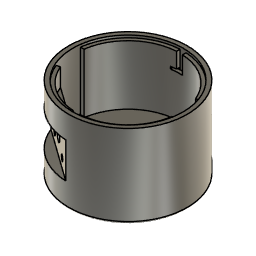
lamp_base v7 (Autodesk Fusion 360 design; units mm, degrees)
Autodesk Fusion 360 part; units mm, degrees
note: some values were not read from the file. Chosen so that the rebuilt part matches the saved one: which face or edge a step refers to. Set by a fixed rule: which sketch regions a step uses.
sketch "Sketch1" plane through (0, 0, 0) normal (0, 0, 1) x (1, 0, 0)
  circle A0 centre (0, 0) radius 50
  constraint coincident A0.centre origin
extrude "Extrude1" add sketch "Sketch1" along normal blind 70
sketch "Sketch2" plane through (0, 0, 0) normal (0, 0, -1) x (1, 0, 0)
  circle A0 centre (0, 0) radius 50
  circle A1 centre (0, 0) radius 40
  dimension "d3" = 80
  constraint coincident A0.centre A1.centre
  measures "d3" diameter of A1
extrude "Extrude2" cut sketch "Sketch2" against normal blind 10 contours A1
sketch "Sketch3" plane through (0, 0, 70) normal (0, 0, 1) x (-1, 0, 0)
  circle A0 centre (0, 0) radius 50
  circle A1 centre (0, 0) radius 46.5
  dimension "d6" = 93
  constraint coincident A0.centre A1.centre
  measures "d6" diameter of A1
extrude "Extrude3" cut sketch "Sketch3" against normal blind 2 contours A1
sketch "Sketch4" plane through (0, 0, 68) normal (0, 0, 1) x (-1, 0, 0)
  circle A0 centre (0, 0) radius 46.5
  circle A1 centre (0, 0) radius 43.5
  dimension "d9" = 87
  constraint coincident A0.centre A1.centre
  measures "d9" diameter of A1
extrude "Extrude4" cut sketch "Sketch4" against normal blind 50 contours A1
sketch "Sketch5" plane through (0, 0, 68) normal (0, 0, 1) x (-1, 0, 0)
  circle A0 centre (0, 0) radius 43.5
  circle A1 centre (0, 0) radius 46.5
  arc A2 (-2.5, -46.4327) -> (2.5, -46.4327) centre (0, 0) ccw
  arc A3 (2.5, 46.4327) -> (-2.5, 46.4327) centre (0, 0) ccw
  line L0 (2.5, 43.4281) -> (-2.5, 43.4281)
  line L1 (2.5, -43.4281) -> (-2.5, -43.4281)
  line L2 (2.5, -46.4327) -> (2.5, -43.4281)
  line L3 (2.5, 43.4281) -> (2.5, 46.4327)
  line L4 (-2.5, 46.4327) -> (-2.5, 43.4281)
  line L5 (-2.5, -43.4281) -> (-2.5, -46.4327)
  dimension "d12" = 5
  constraint coincident A0.centre A1.centre
  constraint vertical L2
  constraint vertical L4
  constraint coincident A3.start A2
  constraint concentric A2 A3
  constraint coincident A0 L0.start
  constraint coincident L0.start L2
  constraint coincident A0 L0.end
  constraint perpendicular L0 L4
  constraint coincident A0 L1.start
  constraint coincident A0 L1.end
  constraint coincident L1.end L4
  constraint collinear L2 L3
  constraint collinear L4 L5
  measures "d12" distance of L2 L4
extrude "Extrude5" cut sketch "Sketch5" against normal blind 15 contours A0 A1 A3 L3 L4 | A0 A1 A2 L2 L5
sketch "Sketch6" plane through (0, 0, 53) normal (0, 0, 1) x (-1, 0, 0)
  line L0 (2.5, 43.4281) -> (2.5, 46.4327)
  arc A0 (2.5, 46.4327) -> (-2.5, 46.4327) centre (0, 0) ccw
  line L1 (-2.5, 46.4327) -> (-2.5, 43.4281)
  arc A1 (2.5, 43.4281) -> (-2.5, 43.4281) centre (0, 0) ccw
  circle A2 centre (0, 0) radius 46.5
  line L2 (-2.5, 46.4327) -> (7.4711, -45.8959)
  line L3 (7.4711, -45.8959) -> (2.5, -46.4327)
  line L4 (2.5, -46.4327) -> (-7.4711, 45.8959)
  line L5 (-7.4711, 45.8959) -> (-2.5, 46.4327)
  dimension "d15" = 93
  dimension "d16" = 5
  constraint concentric A0 A2
  constraint perpendicular L2 L3
  constraint parallel L2 L4
  constraint parallel L3 L5
  constraint coincident A2 L2.end
  constraint coincident A0.end L1.start
  constraint coincident A2 L4.end
  measures "d15" diameter of A2
  measures "d16" distance of L2 L4
extrude "Extrude6" cut sketch "Sketch6" along normal blind 2 contours L1 A1 L2 L3 L4 L5
sketch "Sketch7" plane through (0, 0, 68) normal (0, 0, 1) x (-1, 0, 0)
  line L0 (-2.5, 43.4281) -> (-2.5, 46.4327)
  arc A0 (-2.5, 46.4327) -> (-2.5, -46.4327) centre (0, 0) ccw
  line L1 (-2.5, -46.4327) -> (-2.5, -43.4281)
  arc A1 (-2.5, 43.4281) -> (-2.5, -43.4281) centre (0, 0) ccw
  line L2 (-46.1113, 6) -> (-0.7807, 6)
  line L3 (-43.0404, -17.6004) -> (0.7807, -6)
  line L4 (43.0404, 17.6004) -> (-0.7807, 6)
  line L5 (46.1113, -6) -> (0.7807, -6)
  arc A2 (-46.1113, 6) -> (-43.0404, -17.6004) centre (0, 0) ccw
  arc A3 (46.1113, -6) -> (43.0404, 17.6004) centre (0, 0) ccw
  dimension "d19" = 93
  dimension "d20" = 12
  dimension "d21" = 12
  constraint coincident A0.centre A1.centre
  constraint horizontal L2
  constraint horizontal L5
  constraint coincident L5.start A2
  constraint coincident A0 L2.start
  constraint parallel L3 L4
  constraint coincident L4.start A2
  constraint concentric A2 A3
  measures "d19" diameter of A2
  measures "d20" distance of L2 L5
  measures "d21" distance of L3 L4
extrude "Extrude7" cut sketch "Sketch7" against normal blind 50 contours A1 L2 L3 L4 L5 A3 | A0 A1 L2 L3 A2
sketch "Sketch8" plane through (0, 0, 18) normal (0, 0, 1) x (-1, 0, 0)
  arc A0 (40.1141, 16.8258) -> (-43.0842, 6) centre (0, 0) ccw
  line L0 (-43.0842, 6) -> (-46.1113, 6)
  arc A1 (-46.1113, 6) -> (-43.0404, -17.6004) centre (0, 0) ccw
  line L1 (-43.0404, -17.6004) -> (-40.1141, -16.8258)
  arc A2 (-40.1141, -16.8258) -> (43.0842, -6) centre (0, 0) ccw
  line L2 (43.0842, -6) -> (46.1113, -6)
  arc A3 (46.1113, -6) -> (43.0404, 17.6004) centre (0, 0) ccw
  line L3 (43.0404, 17.6004) -> (40.1141, 16.8258)
fillet "Fillet1" radius 2 1 edges at (-46.6164, -18.0808, 0)
sketch "Sketch11" plane through (0, 0, 68) normal (0, 0, 1) x (-1, 0, 0)
  line L0 (40.1141, 16.8258) -> (43.0404, 17.6004)
  arc A0 (43.0404, 17.6004) -> (2.5, 46.4327) centre (0, 0) ccw
  line L1 (2.5, 46.4327) -> (2.5, 43.4281)
  arc A1 (40.1141, 16.8258) -> (2.5, 43.4281) centre (0, 0) ccw
  line L2 (40.1141, 16.8258) -> (2.5, 43.4281)
  arc A2 (40.1141, 16.8258) -> (2.5, 43.4281) centre (0, 0) ccw
  dimension "d27" = 87
  constraint coincident L0.start A1.start
  constraint coincident L1.end A1.end
  constraint coincident A0.centre A1.centre
  measures "d27" diameter of A2
extrude "Extrude8" add sketch "Sketch11" against normal blind 50 contours A1 L2 A2
sketch "Sketch12" plane through (0, 0, 68) normal (0, 0, 1) x (-1, 0, 0)
  line L0 (40.1141, 16.8258) -> (43.0404, 17.6004)
  arc A0 (43.0404, 17.6004) -> (2.5, 46.4327) centre (0, 0) ccw
  line L1 (2.5, 46.4327) -> (2.5, 43.4281)
  line L2 (2.5, 43.4281) -> (40.1141, 16.8258)
  line L3 (40.1141, 16.8258) -> (46.4504, 18.5031)
  line L4 (2.5, 43.4281) -> (2.5, 49.9375)
  line L5 (46.4504, 18.5031) -> (2.5, 49.9375)
  arc A1 (46.4504, 18.5031) -> (2.5, 49.9375) centre (0, 0) ccw
  dimension "d30" = 100
  constraint concentric A0 A1
  constraint coincident L0.start L2.end
  constraint parallel L0 L3
  constraint coincident L1.end L2.start
  constraint parallel L1 L4
  measures "d30" diameter of A1
extrude "Extrude9" cut sketch "Sketch12" against normal blind 30 from surface at -18 contours A0 L5 | A0 L5 A1
sketch "Sketch13" plane through (0, 0, 68) normal (0, 0, 1) x (-1, 0, 0)
  line L0 (40.1141, 16.8258) -> (43.0404, 17.6004)
  arc A0 (43.0404, 17.6004) -> (2.5, 46.4327) centre (0, 0) ccw
  line L1 (2.5, 46.4327) -> (2.5, 43.4281)
  line L2 (2.5, 43.4281) -> (40.1141, 16.8258)
  circle A1 centre (0, 0) radius 43.5
  line L3 (2.5, 43.4281) -> (40.1141, 16.8258)
  constraint coincident A0.centre A1.centre
  constraint coincident L1.end A1
  constraint coincident L1.end L2.start
  constraint coincident L0.start L2.end
extrude "Extrude10" cut sketch "Sketch13" against normal blind 15 contours L2 A1 L3 | L2 A1 L3
sketch "Sketch14" plane through (0, 0, 0) normal (0, 0, -1) x (1, 0, 0)
  circle A0 centre (0, 0) radius 40
  circle A1 centre (0, 0) radius 48
  circle A2 centre (0, 0) radius 50
  dimension "d36" = 100
  constraint concentric A0 A2
  measures "d36" diameter of A2
sketch "Sketch15" plane through (-24.4752, -34.2203, 0) normal (-0.581744, -0.813372, 0) x (0.813372, -0.581744, 0)
  line L0 (27.0174, 50) -> (-27.0174, 50)
  line L1 (-27.0174, 50) -> (-27.0174, 20)
  line L2 (-27.0174, 20) -> (27.0174, 20)
  line L3 (27.0174, 20) -> (27.0174, 50)
  line L4 (-27.0174, 20) -> (-27.0174, 0)
  line L5 (-27.0174, 0) -> (27.0174, 0)
  line L6 (27.0174, 0) -> (27.0174, 20)
  constraint coincident L1.end L2.start
  constraint perpendicular L2 L4
  constraint perpendicular L3 L5
  constraint coincident L2.end L3.start
  constraint perpendicular L2 L6
sketch "Sketch16" plane through (0, 0, 0) normal (0, 0, -1) x (1, 0, 0)
  line L0 (-46.5152, 18.3394) -> (-2.261, 49.9489)
  line L1 (-2.261, 49.9489) -> (46.5152, -18.3394)
  line L2 (2.261, -49.9489) -> (-46.5152, 18.3394)
  circle A0 centre (0, 0) radius 50
  line L3 (46.5152, -18.3394) -> (29.7583, -30.3084)
  line L4 (19.0179, -37.9799) -> (2.261, -49.9489)
  line L5 (29.7583, -30.3084) -> (43.266, -49.2197)
  line L6 (43.266, -49.2197) -> (32.5257, -56.8912)
  line L7 (32.5257, -56.8912) -> (19.0179, -37.9799)
  line L8 (29.7583, -30.3084) -> (17.998, -13.8436)
  line L9 (17.998, -13.8436) -> (7.2576, -21.5151)
  line L10 (7.2576, -21.5151) -> (19.0179, -37.9799)
  constraint perpendicular L0 L1
  constraint parallel L0 L3
  constraint parallel L1 L2
  constraint coincident L0.start A0
  constraint coincident L0.end A0
  constraint coincident L1.end A0
  constraint collinear L3 L4
  constraint equal L3 L4
  constraint parallel L5 L7
  constraint parallel L8 L10
extrude "Extrude11" cut sketch "Sketch16" against normal blind 10 contours A0 L5 L7 L8 L9 L10 | A0 L5 L6 L7
fillet "Fillet2" radius 2 1 edges at (31.2391, 32.3815, 10)
fillet "Fillet3" radius 2 1 edges at (20.4987, 40.053, 10)
hole "Hole1" at (16.3478, 22.8843, 18) direction (0, 0, -1) diameter 15 depth 20 tip angle 118
sketch "Sketch18" plane through (-24.4752, -34.2203, 0) normal (-0.581744, -0.813372, 0) x (0.813372, -0.581744, 0)
  line L0 (27.0174, 50) -> (-27.0174, 50)
  line L1 (-27.0174, 50) -> (-27.0174, 20)
  line L2 (-27.0174, 20) -> (27.0174, 20)
  line L3 (27.0174, 20) -> (27.0174, 50)
  line L4 (-27.0174, 35) -> (27.0174, 35)
  line L5 (0, 35) -> (0, 20)
  line L6 (0, 27.5) -> (27.0174, 27.5)
  line L7 (13.5087, 27.5) -> (13.5087, 35)
  line L8 (0, 27.5) -> (-27.0174, 27.5)
  line L9 (-27.0174, 27.5) -> (-13.5087, 27.5)
  line L10 (-13.5087, 35) -> (-13.5087, 27.5)
  line L11 (0, 35) -> (0, 50)
  line L12 (0, 42.5) -> (27.0174, 42.5)
  constraint midpoint L1 L4.start
  constraint midpoint L3 L4.end
  constraint midpoint L4 L5.start
  constraint midpoint L2 L5.end
  constraint midpoint L5 L6.start
  constraint coincident L3 L6.end
  constraint perpendicular L3 L6
  constraint midpoint L6 L7.start
  constraint coincident L4 L7.end
  constraint perpendicular L4 L7
  constraint coincident L1 L8.end
  constraint perpendicular L1 L8
  constraint midpoint L8 L9.end
  constraint coincident L4 L10.start
  constraint perpendicular L9 L10
  constraint midpoint L0 L11.end
  constraint midpoint L11 L12.start
  constraint coincident L3 L12.end
  constraint perpendicular L3 L12
hole "Hole6" at (-35.4628, -26.3617, 27.5) direction (0.581744, 0.813372, 0) diameter 5 depth 10 tip angle 118
hole "Hole7" at (-13.4876, -42.0789, 27.5) direction (0.581744, 0.813372, 0) diameter 5 depth 10 tip angle 118
hole "Hole8" at (-24.4752, -34.2203, 35) direction (0.581744, 0.813372, 0) diameter 10 depth 10 tip angle 118
sketch "Sketch19" plane through (0, 0, 18) normal (0, 0, 1) x (-1, 0, 0)
  circle A0 centre (-16.3478, -22.8843) radius 7.5
  line L0 (40.1141, 16.8258) -> (2.5, 43.4281)
  arc A1 (2.5, 43.4281) -> (-43.0842, 6) centre (0, 0) ccw
  line L1 (-43.0842, 6) -> (-46.1113, 6)
  arc A2 (-46.1113, 6) -> (-43.0404, -17.6004) centre (0, 0) ccw
  line L2 (-43.0404, -17.6004) -> (-40.1141, -16.8258)
  arc A3 (-40.1141, -16.8258) -> (43.0842, -6) centre (0, 0) ccw
  line L3 (43.0842, -6) -> (46.1113, -6)
  arc A4 (46.1113, -6) -> (43.0404, 17.6004) centre (0, 0) ccw
  line L4 (43.0404, 17.6004) -> (40.1141, 16.8258)
  circle A5 centre (0, 0) radius 46.5
  circle A6 centre (0, 0) radius 46.5
  line L5 (43.0404, 17.6004) -> (-43.0404, -17.6004)
  line L6 (-46.1113, 6) -> (46.1113, -6)
  constraint coincident A1.centre A2.centre
  constraint coincident A4.end A5
  constraint concentric A5 A6
  constraint coincident A4.end A6
  constraint coincident A4.end L4.start
  constraint coincident A2.end L2.start
  constraint coincident L1.end A2.start
  constraint coincident L3.end A4.start
hole "Hole9" at (0, 0, 18) direction (0, 0, -1) diameter 5 depth 8 tip angle 118
pattern_linear "R-Pattern1" count 2 spacing 10 along (0.816444, -0.577424, 0) of "Hole9"
pattern_linear "R-Pattern2" count 2 spacing 10 along (-0.816444, 0.577424, 0) of "Hole9"
